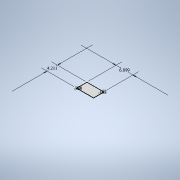
# Autodesk Inventor part: Compute Module Cover for RoadBot Rail-r1
Saved by Autodesk Inventor 2020 (Build 240168000, 168)
## iProperties
Created: 2022-03-30
Part Number: Compute Module Cover for RoadBot Rail-r1
Material: Generic
Document SubType Name: Modeling
Designer: Beaucage
Density: 1 g/cm^3
Appearance: Default
Author: Beaucage
Autodesk Inventor part; units mm, degrees
ref_plane "YZ Plane" through (0, 0, 0) normal (1, 0, 0) x (0, 1, 0)
ref_plane "XZ Plane" through (0, 0, 0) normal (0, 1, 0) x (-1, 0, 0)
ref_plane "XY Plane" through (0, 0, 0) normal (0, 0, 1) x (1, 0, 0)
sketch "Sketch1" plane through (0, 0, 0) normal (0, 1, 0) x (-1, 0, 0)
  line L0 (0, 0) -> (175.2252, 0)
  line L1 (175.2252, 0) -> (175.2252, -106.95)
  line L2 (175.2252, -106.95) -> (0, -106.95)
  line L3 (0, -106.95) -> (0, 0)
  line L4 (0, -106.95) -> (4.2625, -106.95)
  line L5 (4.2625, -106.95) -> (4.2625, -102.6875)
  line L6 (4.2625, -102.6875) -> (0, -102.6875)
  line L7 (0, -102.6875) -> (0, -106.95)
  line L8 (175.2252, 0) -> (170.9627, 0)
  line L9 (170.9627, 0) -> (170.9627, -4.2625)
  line L10 (170.9627, -4.2625) -> (175.2252, -4.2625)
  line L11 (175.2252, -4.2625) -> (175.2252, 0)
  dimension "d0" = 175.2252
  dimension "d1" = 106.95
  dimension "d2" = 4.2625
  dimension "d3" = 4.2625
  dimension "d4" = 4.2625
  dimension "d5" = 4.2625
  constraints: 24 end point, 6 parallel, 3 horizontal, 3 perpendicular
  measures "d0" distance of L1.end L2.end
  measures "d1" distance of L0.end L1.end
  measures "d2" distance of L6.end L5.end
  measures "d3" distance of L5.end L4.end
  measures "d4" distance of L10.end L9.end
  measures "d5" distance of L9.end L8.end
extrude "Extrusion1" add sketch "Sketch1" against normal blind 1.5875
hole "Hole1" at (-170.9627, 0, -4.2625) at (-4.2625, 0, -102.6875) direction (0, -1, 0) diameter 3.2766 end through all clearance for "Flat Head Machine Screw (82)" size "#4" standard "Ansi Unified Screw Threads"
body "Solid1"
